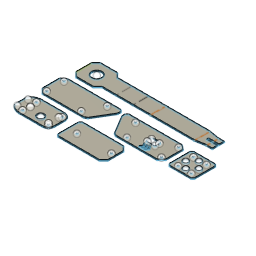
Presenter_Plate (Autodesk Fusion 360 design; units mm, degrees)
part number: 2025-10-11-13-26-14-303
part number: 2025-10-14-21-11-11-009
part number: 2025-10-14-21-11-19-403
part number: 2025-10-14-21-11-23-132
part number: 2025-10-14-21-11-26-400
part number: 2025-10-14-21-11-29-767
part number: 2025-10-14-21-11-34-243
Autodesk Fusion 360 part; units mm, degrees
sketch "スケッチ1" plane through (0, 0, 0) normal (0, 1, 0) x (1, 0, 0)
  circle A0 centre (18, 0) radius 6
  line L0 (8, -14) -> (3, -9)
  line L1 (49, -9) -> (33, -9)
  line L2 (28, -14) -> (8, -14)
  line L3 (33, 9) -> (49, 9)
  line L4 (33, -9) -> (28, -14)
  line L5 (3, 9) -> (8, 14)
  line L6 (49, 9) -> (49, -9) construction
  line L7 (8, 14) -> (28, 14)
  line L8 (3, -9) -> (3, 9)
  line L9 (28, 14) -> (33, 9)
  line L10 (139.6583, -9) -> (89.3799, -9)
  line L11 (89.3799, 9) -> (139.6583, 9)
  line L12 (88.5949, 9) -> (68.625, 9)
  line L13 (88.5949, -9) -> (88.5949, 9) construction
  line L14 (68.625, 9) -> (68.625, -9) construction
  line L15 (68.625, -9) -> (88.5949, -9)
  line L16 (146.5822, 1) -> (151.5822, 1)
  line L17 (146.5822, -1) -> (146.5822, 1)
  line L18 (151.5822, -7) -> (151.5822, -1) construction
  line L19 (151.5822, 1) -> (151.5822, 7) construction
  line L20 (151.5822, 7) -> (139.9883, 9)
  line L21 (139.9883, 9) -> (139.9883, -9) construction
  line L22 (151.5822, -1) -> (146.5822, -1)
  line L23 (139.9883, -9) -> (151.5822, -7)
  line L24 (152.0822, 7) -> (152.0822, 1) construction
  line L25 (158.9419, 7) -> (152.0822, 7)
  line L26 (158.9419, 1) -> (158.9419, 7)
  line L27 (152.0822, 1) -> (158.9419, 1)
  line L28 (152.0822, -1) -> (152.0822, -7) construction
  line L29 (152.0822, -7) -> (158.9419, -7)
  line L30 (158.9419, -1) -> (152.0822, -1)
  line L31 (158.9419, -7) -> (158.9419, -1)
  circle A1 centre (5, -25) radius 1
  circle A2 centre (55, -25) radius 1
  circle A3 centre (5, -45) radius 1
  circle A4 centre (45, -45) radius 1
  line L32 (53, -50) -> (56.029, -48.285)
  line L33 (56.029, -48.285) -> (69, -26.6667)
  line L34 (69, -23) -> (67, -21)
  line L35 (0, -45) -> (5, -50)
  line L36 (5, -50) -> (53, -50)
  line L37 (67, -21) -> (5, -21)
  line L38 (5, -21) -> (0, -25)
  line L39 (69, -26.6667) -> (69, -23)
  line L40 (0, -25) -> (0, -45)
  circle A5 centre (138, -25) radius 1
  circle A6 centre (88, -25) radius 1
  circle A7 centre (138, -45) radius 1
  circle A8 centre (98, -45) radius 1
  line L41 (74, -26.6667) -> (86.971, -48.285)
  line L42 (143, -25) -> (138, -21)
  line L43 (138, -21) -> (76, -21)
  line L44 (138, -50) -> (143, -45)
  line L45 (86.971, -48.285) -> (90, -50)
  line L46 (143, -45) -> (143, -25)
  line L47 (76, -21) -> (74, -23)
  line L48 (74, -23) -> (74, -26.6667)
  line L49 (90, -50) -> (138, -50)
  line L50 (113.58, -31) -> (122.58, -31)
  line L51 (122.58, -38) -> (113.58, -38)
  arc A9 (112.58, -32) -> (113.58, -31) centre (113.58, -32) cw
  line L52 (112.58, -37) -> (112.58, -32)
  arc A10 (123.58, -37) -> (122.58, -38) centre (122.58, -37) cw
  arc A11 (122.58, -31) -> (123.58, -32) centre (122.58, -32) cw
  arc A12 (113.58, -38) -> (112.58, -37) centre (113.58, -37) cw
  line L53 (123.58, -32) -> (123.58, -37)
  line L54 (114, -41) -> (115, -41)
  line L55 (115, -47) -> (114, -47)
  line L56 (114, -47) -> (116, -44.1429)
  line L57 (116, -44.1429) -> (114, -41)
  line L58 (117, -44) -> (115, -47)
  line L59 (115, -41) -> (117, -44)
  line L60 (118, -41) -> (120, -44)
  line L61 (119, -44.1429) -> (117, -41)
  line L62 (117, -47) -> (119, -44.1429)
  line L63 (120, -44) -> (118, -47)
  line L64 (117, -41) -> (118, -41)
  line L65 (118, -47) -> (117, -47)
  line L66 (122, -44.1429) -> (120, -41)
  line L67 (121, -47) -> (120, -47)
  line L68 (123, -44) -> (121, -47)
  line L69 (121, -41) -> (123, -44)
  line L70 (120, -47) -> (122, -44.1429)
  line L71 (120, -41) -> (121, -41)
  circle A13 centre (156.2448, -43.89) radius 1
  circle A14 centre (171.4848, -26.11) radius 1
  circle A15 centre (171.4848, -43.89) radius 1
  circle A16 centre (156.2448, -26.11) radius 1
  circle A17 centre (163.8648, -27.38) radius 3
  circle A18 centre (156.2448, -35) radius 3
  circle A19 centre (163.8648, -42.62) radius 3
  circle A20 centre (171.4848, -35) radius 3
  line L72 (176.4422, -21) -> (151.2875, -21)
  line L73 (149.2875, -47) -> (151.2875, -49)
  line L74 (176.4422, -49) -> (178.4422, -47)
  line L75 (151.2875, -21) -> (149.2875, -23)
  line L76 (149.2875, -23) -> (149.2875, -47)
  line L77 (151.2875, -49) -> (176.4422, -49)
  line L78 (178.4422, -23) -> (176.4422, -21)
  line L79 (178.4422, -47) -> (178.4422, -23)
  circle A21 centre (10, -78) radius 1
  circle A22 centre (40, -62) radius 1
  circle A23 centre (10, -62) radius 1
  circle A24 centre (40, -78) radius 1
  circle A25 centre (27, -74) radius 4
  arc A26 (38, -83) -> (45, -76) centre (38, -76) ccw
  arc A27 (0, -76.3246) -> (0.3636, -77.4745) centre (2, -76.3246) ccw
  arc A28 (45, -64) -> (38, -57) centre (38, -64) ccw
  line L80 (45, -76) -> (45, -64)
  arc A29 (10.9987, -57) -> (0.3636, -62.5255) centre (11, -70) ccw
  arc A30 (0.3636, -77.4745) -> (11.0013, -83) centre (11, -70) ccw
  arc A31 (0.3636, -62.5255) -> (0, -63.6754) centre (2, -63.6754) ccw
  line L81 (0, -63.6754) -> (0, -76.3246)
  line L82 (38, -57) -> (10.9987, -57)
  line L83 (11.0013, -83) -> (38, -83)
  circle A32 centre (65, -70) radius 1
  circle A33 centre (105, -70) radius 1
  line L84 (55, -58) -> (55, -82)
  line L85 (55, -82) -> (57, -84)
  line L86 (57, -84) -> (105, -84)
  line L87 (105, -56) -> (57, -56)
  line L88 (110, -61) -> (105, -56)
  line L89 (110, -79) -> (110, -61)
  line L90 (57, -56) -> (55, -58)
  line L91 (105, -84) -> (110, -79)
  line L92 (49, 9) -> (68.625, 9)
  line L93 (49, -9) -> (68.625, -9)
  line L94 (68.625, 9) -> (68.625, -9) construction
  line L95 (88.5949, 9) -> (89.3799, 9)
  line L96 (89.3799, 9) -> (89.3799, -9) construction
  line L97 (89.3799, -9) -> (88.5949, -9)
  line L98 (88.5949, -9) -> (88.5949, 9) construction
  line L99 (139.6583, 9) -> (139.9883, 9)
  line L100 (139.9883, 9) -> (139.9883, -9) construction
  line L101 (139.9883, -9) -> (139.6583, -9)
  line L102 (139.6583, -9) -> (139.6583, 9) construction
  line L103 (151.5822, 7) -> (152.0822, 7)
  line L104 (152.0822, 7) -> (152.0822, 1) construction
  line L105 (152.0822, 1) -> (151.5822, 1)
  line L106 (151.5822, -1) -> (152.0822, -1)
  line L107 (152.0822, -1) -> (152.0822, -7) construction
  line L108 (152.0822, -7) -> (151.5822, -7)
  dimension "d1" = 19.625
  dimension "d2" = 19.9699
  dimension "d3" = 46
  dimension "d4" = 0.785
  dimension "d5" = 50.2784
  dimension "d6" = 0.33
  dimension "d7" = 0.5
  dimension "d8" = 11.5938
  dimension "d9" = 6.8597
  constraint perpendicular L6 L92
  constraint perpendicular L6 L93
  constraint equal L92 L93
  constraint collinear L14 L94
  constraint horizontal L95
  constraint vertical L96
  constraint horizontal L97
  constraint vertical L98
  constraint horizontal L99
  constraint vertical L100
  constraint horizontal L101
  constraint vertical L102
  constraint collinear L21 L100
  constraint perpendicular L19 L103
  constraint perpendicular L103 L104
  constraint perpendicular L18 L106
  constraint perpendicular L22 L107
  constraint collinear L24 L104
  constraint collinear L28 L107
  measures "d1" distance of L3.end L12.end
  measures "d2" distance of L12.start L12.end
  measures "d3" distance of L6 L8
  measures "d4" distance of L12.start L11.start
  measures "d5" distance of L11.end L11.start
  measures "d6" distance of L11.end L20.end
  measures "d7" distance of L19.end L24.start
  measures "d8" distance of L19 L100
  measures "d9" distance of L26 L104
extrude "押し出し1" add sketch "スケッチ1" along normal blind 1 contours A26 A27 A28 L80 A29 A30 A31 L81 L82 L83 makes body 1
extrude "押し出し2" add sketch "スケッチ1" along normal blind 1 separate body contours L0 L1 L2 L3 L4 L5 L7 L8 L9 L10 L11 L12 L15 L16 L17 L20 L22 L23 L25 L26 L27 L29 L30 L31 L92 L93 L95 L97 L99 L101 L103 L105 L106 L108 | L32 L33 L34 L35 L36 L37 L38 L39 L40 | L41 L42 L43 L44 L45 L46 L47 L48 L49 | L72 L73 L74 L75 L76 L77 L78 L79 | L84 L85 L86 L87 L88 L89 L90 L91 makes body 2 at (99.8519, 0, 33.8122) makes body 3 at (75.8745, 0, 60.4061) makes body 4 at (177.1231, 0, 35) makes body 5 at (34.7922, 0, 31.4061) makes body 6 at (104.3256, 0, 3)
copy_body "ボディ -> コンポーネント1" bodies 1 removing the originals makes body 7 in component "Component"
copy_body "ボディ -> コンポーネント2" bodies 2 removing the originals makes body 8 in component "Component'"
copy_body "ボディ -> コンポーネント3" bodies 3 removing the originals makes body 9 in component "Component''"
copy_body "ボディ -> コンポーネント4" bodies 4 removing the originals makes body 10 in component "Component'''"
copy_body "ボディ -> コンポーネント5" bodies 5 removing the originals makes body 11 in component "Component''''"
copy_body "ボディ -> コンポーネント6" bodies 6 removing the originals makes body 12 in component "Component'''''"
component "Component" placed x (1, 0, 0) y (0, 1, 0) z (0, 0, 1) at (0, 0, 0)
component "Component'" placed x (1, 0, 0) y (0, 1, 0) z (0, 0, 1) at (0, 0, 0)
component "Component''" placed x (1, 0, 0) y (0, 1, 0) z (0, 0, 1) at (0, 0, 0)
component "Component'''" placed x (1, 0, 0) y (0, 1, 0) z (0, 0, 1) at (0, 0, 0)
component "Component''''" placed x (1, 0, 0) y (0, 1, 0) z (0, 0, 1) at (0, 0, 0)
component "Component'''''" placed x (1, 0, 0) y (0, 1, 0) z (0, 0, 1) at (0, 0, 0)
